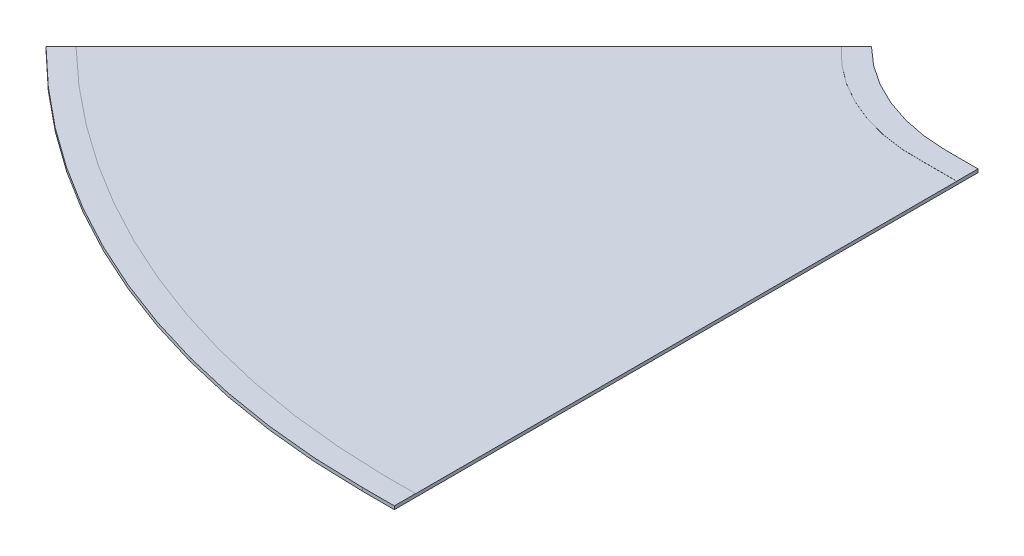
# Autodesk Inventor part: curve_left
Saved by Autodesk Inventor 2021 (Build 250183000, 183)
## iProperties
Created: 2021-01-02
Part Number: curve_left
Material: Generic
Document SubType Name: Modeling
Designer: Tomasz
Density: 1 g/cm^3
Appearance: Default
Author: Tomasz
Autodesk Inventor part; units mm, degrees
ref_plane "YZ Plane" through (0, 0, 0) normal (1, 0, 0) x (0, 1, 0)
ref_plane "XZ Plane" through (0, 0, 0) normal (0, 1, 0) x (-1, 0, 0)
ref_plane "XY Plane" through (0, 0, 0) normal (0, 0, 1) x (1, 0, 0)
sketch "Sketch1" plane through (0, 0, 0) normal (0, 1, 0) x (-1, 0, 0)
  line L0 (30, 275) -> (0, 275)
  line L1 (0, 275) -> (0, -275)
  line L2 (0, -275) -> (30, -275)
  line L3 (30, -275) -> (30, 275)
  line L4 (539.12, 64.1138) -> (150.2089, -324.7926)
  arc A0 (539.12, 64.1138) -> (30, 275) centre (30, -445) ccw
  arc A1 (150.2089, -324.7926) -> (30, -275) centre (30, -445) ccw
  line L5 (0, 255) -> (30, 255)
  line L6 (0, -255) -> (30, -255)
  arc A2 (524.9778, 49.9717) -> (30, 255) centre (21.7353, -464.9526) ccw
  arc A3 (164.3511, -310.6505) -> (30, -255) centre (38.3697, -424.7938) ccw
  point P0 (0, 0)
  point P1 (0, 0)
  dimension "d0" = 30
  dimension "d1" = 550
  dimension "d4" = 550
  dimension "d8" = 539.12
  dimension "d9" = 720
  dimension "d10" = 170
  dimension "d19" = 20
  dimension "d20" = 20
  dimension "d21" = 20
  dimension "d22" = 20
  dimension "d26" = 170
  dimension "d27" = 720
  constraints: 14 end point, 8 point on circle, 6 point on line, 4 centre point, 3 perpendicular, 2 parallel, 1 coincident, 1 concentric, 1 horizontal, 1 midpoint
  measures "d0" distance of L2.end L1.end
  measures "d1" distance of L1.end L0.end
  measures "d4" distance of L4.start L4.end
  measures "d8" horizontal distance of L0.end L4.start
  measures "d9" radius of A0
  measures "d10" radius of A1
  measures "d19" distance of L4.start A2.start
  measures "d20" distance of L0.end L5.start
  measures "d21" distance of L4.end A3.start
  measures "d22" distance of L1.end L6.start
  measures "d26" radius of A3
  measures "d27" radius of A2
extrude "Extrusion1" add sketch "Sketch1" along normal blind 3
extrude "Extrusion2" add sketch "Sketch1" along normal blind 3.1 contours L3 L5 L1 L0 | A0 L4 A2 L3 | A3 L4 A1 L3 | L3 L2 L1 L6
equation "\"d1\" = track_width"
equation "\"d4\" = d1"
equation "\"d19\" = curb_width"
equation "\"d20\" = curb_width"
equation "\"d21\" = curb_width"
equation "\"d22\" = curb_width"
equation "\"d26\" = d10"
equation "\"d27\" = d9"
equation "\"d6\" = track_height"
equation "\"d24\" = track_height + curb_height"
equation "\"track_width\" = 550"
equation "\"curb_width\" = 20"
equation "\"track_height\" = 3"
equation "\"curb_height\" = 0.1"
body "Solid1"
